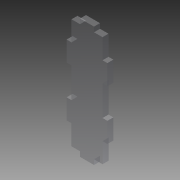
# Autodesk Inventor part: Back_Wall
Saved by Autodesk Inventor 2015 (Build 190159000, 159)
## iProperties
Created: 2015-06-25
Part Number: Back_Wall
Material: Generic
Document SubType Name: Modeling
Designer: Openlab
Density: 1 g/cm^3
Appearance: Polycarbonate - Clear
Author: Openlab
Autodesk Inventor part; units mm, degrees
ref_plane "YZ Plane" through (0, 0, 0) normal (1, 0, 0) x (0, 1, 0)
ref_plane "XZ Plane" through (0, 0, 0) normal (0, 1, 0) x (-1, 0, 0)
ref_plane "XY Plane" through (0, 0, 0) normal (0, 0, 1) x (1, 0, 0)
sketch "Sketch1" plane through (0, 0, 0) normal (0, 1, 0) x (-1, 0, 0)
  line L0 (7.75, -19.9274) -> (7.75, -42.3236) construction
  line L1 (13.2323, -27.5) -> (6.4845, -27.5) construction
  line L2 (15.5, -10) -> (17.95, -10)
  line L3 (17.95, -10) -> (17.95, -20)
  line L4 (17.95, -20) -> (15.5, -20)
  line L5 (15.5, -35) -> (17.95, -35)
  line L6 (17.95, -35) -> (17.95, -45)
  line L7 (17.95, -45) -> (15.5, -45)
  line L8 (0, -10) -> (-2.45, -10)
  line L9 (-2.45, -10) -> (-2.45, -20)
  line L10 (-2.45, -20) -> (0, -20)
  line L11 (0, -35) -> (-2.45, -35)
  line L12 (-2.45, -45) -> (0, -45)
  line L13 (-2.45, -45) -> (-2.45, -35)
  line L14 (15.5, -10) -> (15.5, 0)
  line L15 (15.5, -55) -> (15.5, -45)
  line L16 (15.5, -35) -> (15.5, -20)
  line L17 (0, 0) -> (0, -10)
  line L18 (0, -20) -> (0, -35)
  line L19 (0, -45) -> (0, -55)
  line L20 (4.25, 0) -> (0, 0)
  line L21 (0, -55) -> (4.25, -55)
  line L22 (11.25, -55) -> (15.5, -55)
  line L23 (4.25, 0) -> (4.25, 2.45)
  line L24 (4.25, 2.45) -> (11.25, 2.45)
  line L25 (11.25, 2.45) -> (11.25, 0)
  line L26 (11.25, 0) -> (15.5, 0)
  line L27 (11.25, -55) -> (11.25, -57.45)
  line L28 (11.25, -57.45) -> (4.25, -57.45)
  line L29 (4.25, -57.45) -> (4.25, -55)
  dimension "d8" = 10
  dimension "d9" = 15
  dimension "d10" = 15.5
  dimension "d17" = 2.45
  dimension "d19" = 7
  dimension "d20" = 55
  constraints: 60 end point, 17 perpendicular, 12 parallel, 9 collinear, 8 point on line, 4 equal length, 4 horizontal, 3 vertical, 1 coincident, 5 other
  measures "d8" distance of L2.end L3.end
  measures "d9" distance between parallel lines of L5 L4
  measures "d10" distance between parallel lines of L19 L15
  measures "d17" distance of L8.start L8.end
  measures "d19" distance of L23.end L24.end
  measures "d20" distance between parallel lines of L22 L26
extrude "Extrusion1" add sketch "Sketch1" along normal blind 3
body "Solid1"
